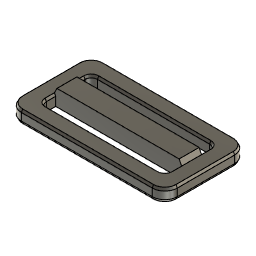
NG_2-3_CAD (Autodesk Fusion 360 design; units mm, degrees)
Autodesk Fusion 360 part; units mm, degrees
note: some values were not read from the file. Chosen so that the rebuilt part matches the saved one: a side; which pieces of a blend or face edit are solid.
sketch "Sketch1" plane through (0, 0, 0) normal (0, 0, 1) x (1, 0, 0)
  line L0 (4, 0) -> (46, 0) construction
  line L1 (50, 0) -> (50, 22.4) construction
  line L2 (50, 26.4) -> (0, 26.4) construction
  line L3 (0, 22.4) -> (0, 0) construction
  line L4 (0, 13.2) -> (50, 13.2) construction
  line L5 (0, 16.4) -> (50, 16.4)
  line L6 (50, 16.4) -> (50, 13.2)
  line L7 (50, 13.2) -> (0, 13.2)
  line L8 (0, 13.2) -> (0, 16.4)
  line L9 (4, 26.4) -> (46, 26.4)
  line L10 (50, 26.4) -> (50, 4)
  line L11 (50, 0) -> (0, 0)
  line L12 (0, 4) -> (0, 26.4)
  line L13 (7, 5) -> (43, 5)
  line L14 (45, 7) -> (45, 19.4)
  line L15 (43, 21.4) -> (7, 21.4)
  line L16 (5, 19.4) -> (5, 7)
  line L17 (0, 10) -> (50, 10)
  arc A0 (4, 26.4) -> (0, 22.4) centre (4, 22.4) ccw
  arc A1 (0, 4) -> (4, 0) centre (4, 4) ccw
  arc A2 (46, 0) -> (50, 4) centre (46, 4) ccw
  arc A3 (50, 22.4) -> (46, 26.4) centre (46, 22.4) ccw
  arc A4 (7, 21.4) -> (5, 19.4) centre (7, 19.4) ccw
  arc A5 (5, 7) -> (7, 5) centre (7, 7) ccw
  arc A6 (43, 5) -> (45, 7) centre (43, 7) ccw
  arc A7 (45, 19.4) -> (43, 21.4) centre (43, 19.4) ccw
  line L18 (4.2, 16.4) -> (4.2, 10)
  line L19 (45.8, 16.4) -> (45.8, 10)
  point P0 (0, 13.2)
  dimension "d3" = 3.2
  dimension "d5" = 4
  dimension "d6" = 2
  dimension "d11" = 5
  dimension "d13" = 5
  dimension "d14" = 5
  dimension "d15" = 5
  dimension "d16" = 5
  dimension "d17" = 5
  dimension "d18" = 40
  dimension "d24" = 0.8
  dimension "d26" = 0.8
  constraint horizontal L0
  constraint vertical L1
  constraint horizontal L2
  constraint vertical L3
  constraint coincident L3.end L11.end
  constraint coincident P0 L4.start
  constraint horizontal L5
  constraint vertical L6
  constraint horizontal L7
  constraint vertical L8
  constraint coincident L3 L5.start
  constraint horizontal L9
  constraint vertical L10
  constraint horizontal L11
  constraint vertical L12
  constraint symmetric L4 L5.start L17.start
  constraint symmetric L4 L5.end L17.end
  constraint parallel L0 L13
  constraint parallel L1 L14
  constraint parallel L2 L15
  constraint parallel L3 L16
  constraint coincident L3 P0
  constraint coincident L2.end L9
  constraint coincident L2.end L3
  constraint tangent L9 A0
  constraint tangent L3 A0
  constraint coincident L3.end L12
  constraint coincident L3.end L0
  constraint tangent L12 A1
  constraint tangent L0 A1
  constraint equal A0 A1
  constraint coincident L1.start L0
  constraint coincident L1.start L10
  constraint tangent L0 A2
  constraint tangent L10 A2
  constraint equal A0 A2
  constraint coincident L1 L4.end
  constraint coincident L2.start L1
  constraint coincident L2.start L9
  constraint tangent L1 A3
  constraint tangent L9 A3
  constraint equal A0 A3
  constraint tangent L15 A4
  constraint tangent L16 A4
  constraint tangent L16 A5
  constraint tangent L13 A5
  constraint equal A4 A5
  constraint tangent L13 A6
  constraint tangent L14 A6
  constraint equal A4 A6
  constraint tangent L14 A7
  constraint tangent L15 A7
  constraint equal A4 A7
  constraint horizontal L17
  constraint coincident L5 L18.start
  constraint coincident L17 L18.end
  constraint perpendicular L17 L18
  constraint coincident L5 L19.start
  constraint coincident L17 L19.end
  constraint perpendicular L17 L19
  measures "d3" distance of L5 L7
  measures "d5" radius of A0
  measures "d6" radius of A4
  measures "d11" distance of L10 L14
  measures "d13" distance of L12 L16
  measures "d14" distance of L9 L15
  measures "d15" distance of L11 L13
  measures "d16" distance of L5 L15
  measures "d17" distance of L13 L17
  measures "d18" distance of L14 L16
  measures "d24" distance of L16 L18
  measures "d26" distance of L14 L19
extrude "Extrude1" add sketch "Sketch1" along normal blind 4 contours L5 L9 L10 L12 L14 L15 L16 A0 A3 A4 A7 | L5 L7 L8 L12 L18 | L5 L7 L16 L18 | L7 L12 L17 L18 | L5 L7 L14 L16 | L7 L16 L17 L18 | L10 L11 L12 L13 L14 L16 L17 A1 A2 A5 A6 | L5 L7 L14 L19 | L7 L14 L16 L17 | L5 L6 L7 L10 L19 | L7 L14 L17 L19 | L7 L10 L17 L19
chamfer "Chamfer1" distance 0.4 distance2 0.8 38 edges at (44.4142, 20.8142, 0) (25, 21.4, 0) (5.5858, 20.8142, 0) (5, 17.9, 0) (45, 17.9, 0) (25, 5, 0) (44.4142, 5.5858, 0) (45, 8.5, 0) (5, 8.5, 0) (5.5858, 5.5858, 0) (25, 0, 0) (1.1716, 1.1716, 0) (0, 13.2, 0) (1.1716, 25.2284, 0) (25, 26.4, 0) (48.8284, 25.2284, 0) (50, 13.2, 0) (48.8284, 1.1716, 0) (25, 0, 4) (48.8284, 1.1716, 4) (50, 13.2, 4) (48.8284, 25.2284, 4) (25, 26.4, 4) (1.1716, 25.2284, 4) (0, 13.2, 4) (1.1716, 1.1716, 4) (25, 21.4, 4) (5.5858, 20.8142, 4) (5, 17.9, 4) (45, 17.9, 4) (44.4142, 20.8142, 4) (25, 5, 4) (44.4142, 5.5858, 4) (45, 8.5, 4) (5, 8.5, 4) (5.5858, 5.5858, 4) (25, 10, 0) (25, 16.4, 0) measured on face at (18.3333, 12.1333, 0) measured on face at (18.3333, 12.1333, 0) measured on face at (18.3333, 12.1333, 0) measured on face at (18.3333, 12.1333, 0) measured on face at (18.3333, 12.1333, 0) measured on face at (18.3333, 12.1333, 0) measured on face at (18.3333, 12.1333, 0) measured on face at (18.3333, 12.1333, 0) measured on face at (18.3333, 12.1333, 0) measured on face at (18.3333, 12.1333, 0) measured on face at (32, 0, 1.3333) measured on face at (18.3333, 12.1333, 0) measured on face at (0, 11.0667, 2.6667) measured on face at (18.3333, 12.1333, 0) measured on face at (18, 26.4, 1.3333) measured on face at (18.3333, 12.1333, 0) measured on face at (50, 12.1333, 1.3333) measured on face at (18.3333, 12.1333, 0) measured on face at (32, 0, 1.3333) measured on face at (46.943, 0.1128, 2.6667) measured on face at (50, 12.1333, 1.3333) measured on face at (49.4641, 24.4, 2.6667) measured on face at (18, 26.4, 1.3333) measured on face at (0.22, 23.7083, 2.6667) measured on face at (0, 11.0667, 2.6667) measured on face at (2.1671, 0.4447, 2.6667) measured on face at (31, 21.4, 1.3333) measured on face at (5.0023, 19.4952, 2.6667) measured on face at (5, 18.4, 1.3333) measured on face at (45, 17.4, 1.3333) measured on face at (43.0952, 21.3977, 2.6667) measured on face at (19, 5, 1.3333) measured on face at (43.0952, 5.0023, 1.3333) measured on face at (45, 8, 1.3333) measured on face at (5, 9, 1.3333) measured on face at (5.1433, 6.2567, 2.6667) measured on face at (18.3333, 12.1333, 0) measured on face at (18.3333, 12.1333, 0)
extrude "Extrude2" add sketch "Sketch1" along normal blind 1.6 from surface at 4 contours L5 L7 L14 L16 | L7 L14 L16 L17
chamfer "Chamfer2" distance 0.4 distance2 0.8 4 edges at (45, 13.2, 4) (5, 13.2, 4) (5, 13.2, 5.6) (45, 13.2, 5.6) measured on face at (19, 24.6, 4) measured on face at (19, 24.6, 4) measured on face at (18.3333, 14.2667, 5.6) measured on face at (18.3333, 14.2667, 5.6)
equation "d3 = ( 6.4 / 2 ) * 1 mm"
equation "d7 = Товщина"
equation "d10 = Bevel_Horizontal"
equation "d11 = Товщинарамки"
equation "d13 = d11"
equation "d14 = d11"
equation "d15 = d11"
equation "d16 = d14"
equation "d17 = d14"
equation "d18 = Ширинастропи"
equation "Ширинастропи = 40 mm"
equation "Висота = 4 mm"
equation "d24 = Bevel_Horizontal"
equation "Bevel_Horizontal = 0.8 mm"
equation "d26 = Bevel_Horizontal"
equation "d28 = Bevel_Horizontal"
equation "Товщинарамки = 5 mm"
named bodies: "Ramka"
